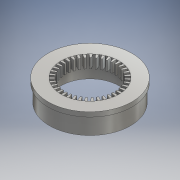
# Autodesk Inventor part: UR5 Wrist Rotation
Saved by Autodesk Inventor 2016 (Build 200138000, 138)
## iProperties
Created: 2017-12-25
Part Number: UR5 Wrist Rotation
Material: Aluminum 6061-AHC
Document SubType Name: Modeling
Designer: kornbot
Density: 2.7 g/cm^3
Appearance: Aluminum - Dark
Author: kornbot
Autodesk Inventor part; units mm, degrees
ref_plane "YZ Plane" through (0, 0, 0) normal (1, 0, 0) x (0, 1, 0)
ref_plane "XZ Plane" through (0, 0, 0) normal (0, 1, 0) x (-1, 0, 0)
ref_plane "XY Plane" through (0, 0, 0) normal (0, 0, 1) x (1, 0, 0)
sketch "Sketch1" plane through (0, 0, 0) normal (0, 0, 1) x (1, 0, 0)
  circle A0 centre (0, 0) radius 25.5
  circle A1 centre (0, 0) radius 35.6825
  dimension "d0" = 51
  dimension "d1" = 71.365
  constraints: 2 centre point, 2 coincident
  measures "d0" diameter of A0
  measures "d1" diameter of A1
extrude "Extrusion1" add sketch "Sketch1" along normal blind 19
sketch "Sketch2" plane through (0, 0, 19) normal (0, 0, 1) x (1, 0, 0)
  circle A0 centre (0, 0) radius 37
  circle A1 centre (0, 0) radius 35.6825
  dimension "d4" = 74
  constraints: 2 centre point, 2 coincident
  measures "d4" diameter of A0
extrude "Extrusion2" add sketch "Sketch2" against normal blind 4
sketch "Sketch3" plane through (0, 0, 19) normal (0, 0, 1) x (1, 0, 0)
  line L0 (-25.465862, -0.020576) -> (-21.481701, -0.020576)
  circle A0 centre (0, 0) radius 32.249031
  line L1 (-21.481701, -0.020576) -> (-21.481701, 0.604424)
  line L2 (-21.481701, -0.06479) -> (-21.481701, -0.68979)
  line L3 (-21.481701, -0.68979) -> (-25.479335, -1.026389)
  circle A1 centre (0, 0) radius 25.5
  line L4 (-21.481701, 0.604424) -> (-25.479335, 1.073894)
  line L5 (-25.479335, 1.073894) -> (-25.479335, -1.026389)
  line L6 (-25.479335, 1.073894) -> (-21.481701, 0.604424)
  line L7 (-21.481701, 0.604424) -> (-21.481701, -0.68979)
  line L8 (-21.481701, -0.68979) -> (-25.479335, -1.026389)
  line L9 (-25.479335, 1.073894) -> (-25.479335, -1.026389)
  line L10 (-25.479335, -1.026389) -> (-21.481701, -0.68979)
  line L11 (-21.481701, -0.68979) -> (-21.481701, 0.604424)
  line L12 (-21.481701, 0.604424) -> (-25.479335, 1.073894)
  line L13 (-21.300475, -2.849311) -> (-25.321649, -3.027185)
  line L14 (-21.200218, -3.466217) -> (-21.300475, -2.849311)
  line L15 (-21.300475, -2.849311) -> (-21.092869, -4.126765)
  line L16 (-21.092869, -4.126765) -> (-24.98474, -5.10027)
  line L17 (-25.321649, -3.027185) -> (-24.98474, -5.10027)
  line L18 (-20.567578, -6.229249) -> (-24.508146, -7.049862)
  line L19 (-20.369661, -6.822085) -> (-20.567578, -6.229249)
  line L20 (-20.567578, -6.229249) -> (-20.157742, -7.456858)
  line L21 (-20.157742, -7.456858) -> (-23.843054, -9.042057)
  line L22 (-24.508146, -7.049862) -> (-23.843054, -9.042057)
  line L23 (-19.301991, -9.447854) -> (-23.059894, -10.889951)
  line L24 (-19.011539, -10.001264) -> (-19.301991, -9.447854)
  line L25 (-19.301991, -9.447854) -> (-18.70054, -10.593823)
  line L26 (-18.70054, -10.593823) -> (-22.083844, -12.74966)
  line L27 (-23.059894, -10.889951) -> (-22.083844, -12.74966)
  line L28 (-17.536493, -12.421764) -> (-21.014404, -14.447997)
  line L29 (-17.161029, -12.921416) -> (-17.536493, -12.421764)
  line L30 (-17.536493, -12.421764) -> (-16.759005, -13.456414)
  line L31 (-16.759005, -13.456414) -> (-19.752675, -16.127053)
  line L32 (-21.014404, -14.447997) -> (-19.752675, -16.127053)
  line L33 (-15.316809, -15.073957) -> (-18.424651, -17.631846)
  line L34 (-14.866058, -15.506909) -> (-15.316809, -15.073957)
  line L35 (-15.316809, -15.073957) -> (-14.383419, -15.97049)
  line L36 (-14.383419, -15.97049) -> (-16.909922, -19.086763)
  line L37 (-18.424651, -17.631846) -> (-16.909922, -19.086763)
  line L38 (-12.700428, -17.335742) -> (-15.35771, -20.35904)
  line L39 (-12.186063, -17.690782) -> (-12.700428, -17.335742)
  line L40 (-12.700428, -17.335742) -> (-11.635311, -18.070939)
  line L41 (-11.635311, -18.070939) -> (-13.629211, -21.552137)
  line L42 (-15.35771, -20.35904) -> (-13.629211, -21.552137)
  line L43 (-9.755112, -19.14854) -> (-11.893012, -22.558946)
  line L44 (-9.190456, -19.416473) -> (-9.755112, -19.14854)
  line L45 (-9.755112, -19.14854) -> (-8.585854, -19.70336)
  line L46 (-8.585854, -19.70336) -> (-9.99551, -23.459322)
  line L47 (-11.893012, -22.558946) -> (-9.99551, -23.459322)
  line L48 (-6.557144, -20.465402) -> (-8.120291, -24.174587)
  line L49 (-5.95682, -20.639288) -> (-6.557144, -20.465402)
  line L50 (-6.557144, -20.465402) -> (-5.314029, -20.825475)
  line L51 (-5.314029, -20.825475) -> (-6.102931, -24.758922)
  line L52 (-8.120291, -24.174587) -> (-6.102931, -24.758922)
  line L53 (-3.18935, -21.25222) -> (-4.137259, -25.164119)
  line L54 (-2.568907, -21.327556) -> (-3.18935, -21.25222)
  line L55 (-3.18935, -21.25222) -> (-1.904572, -21.40822)
  line L56 (-1.904572, -21.40822) -> (-2.052289, -25.41728)
  line L57 (-4.137259, -25.164119) -> (-2.052289, -25.41728)
  line L58 (0.261048, -21.488617) -> (-0.047074, -25.501913)
  line L59 (0.885541, -21.463451) -> (0.261048, -21.488617)
  line L60 (0.261048, -21.488617) -> (1.554212, -21.436504)
  line L61 (1.554212, -21.436504) -> (2.051506, -25.417343)
  line L62 (-0.047074, -25.501913) -> (2.051506, -25.417343)
  line L63 (3.704684, -21.16847) -> (4.04433, -25.179221)
  line L64 (4.317053, -21.043454) -> (3.704684, -21.16847)
  line L65 (3.704684, -21.16847) -> (4.972742, -20.909594)
  line L66 (4.972742, -20.909594) -> (6.102168, -24.75911)
  line L67 (4.04433, -25.179221) -> (6.102168, -24.75911)
  line L68 (7.05237, -20.300071) -> (8.030988, -24.2044)
  line L69 (7.636756, -20.078443) -> (7.05237, -20.300071)
  line L70 (7.05237, -20.300071) -> (8.262481, -19.841137)
  line L71 (8.262481, -19.841137) -> (9.994787, -23.45963)
  line L72 (8.030988, -24.2044) -> (9.994787, -23.45963)
  line L73 (10.217404, -18.905911) -> (11.809648, -22.602699)
  line L74 (10.75867, -18.593411) -> (10.217404, -18.905911)
  line L75 (10.217404, -18.905911) -> (11.338226, -18.258804)
  line L76 (11.338226, -18.258804) -> (13.628546, -21.552557)
  line L77 (11.809648, -22.602699) -> (13.628546, -21.552557)
  line L78 (13.117813, -17.022097) -> (15.282444, -20.415599)
  line L79 (13.601941, -16.626819) -> (13.117813, -17.022097)
  line L80 (13.117813, -17.022097) -> (14.120317, -16.203578)
  line L81 (14.120317, -16.203578) -> (16.909334, -19.087285)
  line L82 (15.282444, -20.415599) -> (16.909334, -19.087285)
  line L83 (15.678477, -14.69742) -> (18.359433, -17.699746)
  line L84 (16.092929, -14.229601) -> (15.678477, -14.69742)
  line L85 (15.678477, -14.69742) -> (16.5367, -13.728688)
  line L86 (16.5367, -13.728688) -> (19.752178, -16.127661)
  line L87 (18.359433, -17.699746) -> (19.752178, -16.127661)
  line L88 (17.833077, -11.992088) -> (20.960922, -14.525479)
  line L89 (18.167118, -11.463844) -> (17.833077, -11.992088)
  line L90 (17.833077, -11.992088) -> (18.52479, -10.898231)
  line L91 (18.52479, -10.898231) -> (22.083451, -12.75034)
  line L92 (20.960922, -14.525479) -> (22.083451, -12.75034)
  line L93 (19.52581, -8.976167) -> (23.019534, -10.975009)
  line L94 (19.770789, -8.40118) -> (19.52581, -8.976167)
  line L95 (19.52581, -8.976167) -> (20.033098, -7.785517)
  line L96 (20.033098, -7.785517) -> (23.842775, -9.042792)
  line L97 (23.019534, -10.975009) -> (23.842775, -9.042792)
  line L98 (20.712834, -5.727768) -> (24.481952, -7.140293)
  line L99 (20.862406, -5.120929) -> (20.712834, -5.727768)
  line L100 (20.712834, -5.727768) -> (21.02256, -4.471162)
  line L101 (21.02256, -4.471162) -> (24.984583, -5.10104)
  line L102 (24.481952, -7.140293) -> (24.984583, -5.10104)
  line L103 (21.363407, -2.331022) -> (25.310301, -3.120647)
  line L104 (21.413698, -1.708049) -> (21.363407, -2.331022)
  line L105 (21.363407, -2.331022) -> (21.467548, -1.041005)
  line L106 (21.467548, -1.041005) -> (25.479304, -1.027174)
  line L107 (25.310301, -3.120647) -> (25.479304, -1.027174)
  line L108 (21.460679, 1.126095) -> (25.483126, 0.979823)
  line L109 (21.410387, 1.749069) -> (21.460679, 1.126095)
  line L110 (21.460679, 1.126095) -> (21.356538, 2.416112)
  line L111 (21.356538, 2.416112) -> (25.314124, 3.073295)
  line L112 (25.483126, 0.979823) -> (25.314124, 3.073295)
  line L113 (21.00213, 4.554047) -> (24.995952, 5.054915)
  line L114 (20.852558, 5.160886) -> (21.00213, 4.554047)
  line L115 (21.00213, 4.554047) -> (20.692404, 5.810654)
  line L116 (20.692404, 5.810654) -> (24.493321, 7.094168)
  line L117 (24.995952, 5.054915) -> (24.493321, 7.094168)
  line L118 (19.999637, 7.864052) -> (23.861395, 8.999088)
  line L119 (19.754658, 8.43904) -> (19.999637, 7.864052)
  line L120 (19.999637, 7.864052) -> (19.492349, 9.054702)
  line L121 (19.492349, 9.054702) -> (23.038155, 10.931305)
  line L122 (23.861395, 8.999088) -> (23.038155, 10.931305)
  line L123 (18.479165, 10.970382) -> (22.108841, 12.710189)
  line L124 (18.145123, 11.498626) -> (18.479165, 10.970382)
  line L125 (18.479165, 10.970382) -> (17.787452, 12.064239)
  line L126 (17.787452, 12.064239) -> (20.986312, 14.485328)
  line L127 (22.108841, 12.710189) -> (20.986312, 14.485328)
  line L128 (16.480091, 13.792585) -> (19.78368, 16.092103)
  line L129 (16.06564, 14.260404) -> (16.480091, 13.792585)
  line L130 (16.480091, 13.792585) -> (15.621869, 14.761318)
  line L131 (15.621869, 14.761318) -> (18.390935, 17.664188)
  line L132 (19.78368, 16.092103) -> (18.390935, 17.664188)
  line L133 (14.054192, 16.257567) -> (16.946131, 19.05724)
  line L134 (13.570064, 16.652846) -> (14.054192, 16.257567)
  line L135 (14.054192, 16.257567) -> (13.051688, 17.076087)
  line L136 (13.051688, 17.076087) -> (15.319242, 20.385554)
  line L137 (16.946131, 19.05724) -> (15.319242, 20.385554)
  line L138 (11.264297, 18.301487) -> (13.669687, 21.528805)
  line L139 (10.723031, 18.613987) -> (11.264297, 18.301487)
  line L140 (11.264297, 18.301487) -> (10.143475, 18.948594)
  line L141 (10.143475, 18.948594) -> (11.850789, 22.578946)
  line L142 (13.669687, 21.528805) -> (11.850789, 22.578946)
  line L143 (8.182662, 19.871408) -> (10.039205, 23.442784)
  line L144 (7.598277, 20.093036) -> (8.182662, 19.871408)
  line L145 (8.182662, 19.871408) -> (6.972551, 20.330342)
  line L146 (6.972551, 20.330342) -> (8.075407, 24.187555)
  line L147 (10.039205, 23.442784) -> (8.075407, 24.187555)
  line L148 (4.889101, 20.92667) -> (6.148713, 24.749608)
  line L149 (4.276732, 21.051686) -> (4.889101, 20.92667)
  line L150 (4.889101, 20.92667) -> (3.621042, 21.185546)
  line L151 (3.621042, 21.185546) -> (4.090876, 25.169719)
  line L152 (6.148713, 24.749608) -> (4.090876, 25.169719)
  line L153 (1.468914, 21.439942) -> (2.098973, 25.41543)
  line L154 (0.844421, 21.465108) -> (1.468914, 21.439942)
  line L155 (1.468914, 21.439942) -> (0.17575, 21.492055)
  line L156 (0.17575, 21.492055) -> (0.000393, 25.5)
  line L157 (2.098973, 25.41543) -> (0.000393, 25.5)
  line L158 (-1.989316, 21.397931) -> (-2.00513, 25.423006)
  line L159 (-2.609759, 21.322595) -> (-1.989316, 21.397931)
  line L160 (-1.989316, 21.397931) -> (-3.274094, 21.24193)
  line L161 (-3.274094, 21.24193) -> (-4.0901, 25.169845)
  line L162 (-2.00513, 25.423006) -> (-4.0901, 25.169845)
  line L163 (-5.396025, 20.801724) -> (-6.057301, 24.772139)
  line L164 (-5.996348, 20.627838) -> (-5.396025, 20.801724)
  line L165 (-5.396025, 20.801724) -> (-6.63914, 20.441651)
  line L166 (-6.63914, 20.441651) -> (-8.074661, 24.187804)
  line L167 (-6.057301, 24.772139) -> (-8.074661, 24.187804)
  line L168 (-8.662979, 19.666764) -> (-9.952591, 23.479687)
  line L169 (-9.227635, 19.398831) -> (-8.662979, 19.666764)
  line L170 (-8.662979, 19.666764) -> (-9.832237, 19.111944)
  line L171 (-9.832237, 19.111944) -> (-11.850093, 22.579311)
  line L172 (-9.952591, 23.479687) -> (-11.850093, 22.579311)
  line L173 (-11.705566, 18.022445) -> (-13.590115, 21.579123)
  line L174 (-12.219931, 17.667405) -> (-11.705566, 18.022445)
  line L175 (-11.705566, 18.022445) -> (-12.770683, 17.287248)
  line L176 (-12.770683, 17.287248) -> (-15.318614, 20.386027)
  line L177 (-13.590115, 21.579123) -> (-15.318614, 20.386027)
  line L178 (-14.444986, 15.911354) -> (-16.875661, 19.119672)
  line L179 (-14.895737, 15.478402) -> (-14.444986, 15.911354)
  line L180 (-14.444986, 15.911354) -> (-15.378376, 15.014821)
  line L181 (-15.378376, 15.014821) -> (-18.39039, 17.664754)
  line L182 (-16.875661, 19.119672) -> (-18.39039, 17.664754)
  line L183 (-16.810288, 13.388168) -> (-19.724137, 16.16503)
  line L184 (-17.185752, 12.888516) -> (-16.810288, 13.388168)
  line L185 (-16.810288, 13.388168) -> (-17.587777, 12.353518)
  line L186 (-17.587777, 12.353518) -> (-20.985865, 14.485974)
  line L187 (-19.724137, 16.16503) -> (-20.985865, 14.485974)
  line L188 (-18.740212, 10.518235) -> (-22.061767, 12.791724)
  line L189 (-19.030664, 9.964825) -> (-18.740212, 10.518235)
  line L190 (-18.740212, 10.518235) -> (-19.341663, 9.372266)
  line L191 (-19.341663, 9.372266) -> (-23.037818, 10.932015)
  line L192 (-22.061767, 12.791724) -> (-23.037818, 10.932015)
  line L193 (-20.184775, 7.375885) -> (-23.82801, 9.087118)
  line L194 (-20.382692, 6.78305) -> (-20.184775, 7.375885)
  line L195 (-20.184775, 7.375885) -> (-20.594611, 6.148276)
  line L196 (-20.594611, 6.148276) -> (-24.493103, 7.094923)
  line L197 (-23.82801, 9.087118) -> (-24.493103, 7.094923)
  line L198 (-21.106562, 4.042504) -> (-24.97712, 5.14716)
  line L199 (-21.206819, 3.425597) -> (-21.106562, 4.042504)
  line L200 (-21.106562, 4.042504) -> (-21.314169, 2.76505)
  line L201 (-21.314169, 2.76505) -> (-25.314029, 3.074075)
  line L202 (-24.97712, 5.14716) -> (-25.314029, 3.074075)
  point P0 (-21.193126, -3.509858)
  point P1 (-20.355659, -6.864023)
  point P2 (-18.990992, -10.040413)
  point P3 (-17.134468, -12.956762)
  point P4 (-14.834171, -15.537537)
  point P5 (-12.149676, -17.715898)
  point P6 (-9.150511, -19.435427)
  point P7 (-5.914352, -20.651589)
  point P8 (-2.525015, -21.332885)
  point P9 (0.929718, -21.461671)
  point P10 (4.360373, -21.03461)
  point P11 (7.678096, -20.062765)
  point P12 (10.79696, -18.571304)
  point P13 (13.636189, -16.598856)
  point P14 (16.122248, -14.196507)
  point P15 (18.190749, -11.426475)
  point P16 (19.788119, -8.360504)
  point P17 (20.872987, -5.078)
  point P18 (21.417256, -1.663979)
  point P19 (21.406829, 1.793139)
  point P20 (20.841977, 5.203815)
  point P21 (19.737328, 8.479715)
  point P22 (18.121493, 11.535995)
  point P23 (16.03632, 14.293499)
  point P24 (13.535816, 16.680809)
  point P25 (10.684741, 18.636094)
  point P26 (7.556936, 20.108714)
  point P27 (4.233411, 21.06053)
  point P28 (0.800243, 21.466888)
  point P29 (-2.653651, 21.317266)
  point P30 (-6.038816, 20.615537)
  point P31 (-9.26758, 19.379877)
  point P32 (-12.256318, 17.642289)
  point P33 (-14.927624, 15.447774)
  point P34 (-17.212313, 12.85317)
  point P35 (-19.051211, 9.925676)
  point P36 (-20.396693, 6.741111)
  point P37 (-21.213912, 3.381956)
  dimension "d13" = 0.625
  dimension "d14" = 0.625
  dimension "d17" = 360
  constraints: 406 end point, 78 point on line, 5 collinear, 2 vertical, 1 centre point, 1 coincident, 1 horizontal, 432 other
  measures "d13" distance of L0.end L1.end
  measures "d14" distance of L2.start L2.end
sketch "Sketch3 outline for Extrusion3" plane through (0, 0, 19) normal (0, 0, 1) x (1, 0, 0)
  circle A0 centre (0, 0) radius 32.249031
  arc A1 (25.314124, -3.073295) -> (25.479304, -1.027174) centre (0, 0) ccw
  line L0 (25.314124, -3.073295) -> (25.479304, -1.027174)
  line L1 (25.479304, -1.027174) -> (21.467548, -1.041005)
  line L2 (21.467548, -1.041005) -> (21.363407, -2.331022)
  line L3 (21.363407, -2.331022) -> (25.308377, -3.120262)
  arc A2 (24.984583, -5.10104) -> (25.308377, -3.120262) centre (0, 0) ccw
  line L4 (24.984583, -5.10104) -> (21.02256, -4.471162)
  line L5 (21.02256, -4.471162) -> (20.712834, -5.727768)
  line L6 (20.712834, -5.727768) -> (24.480115, -7.139604)
  arc A3 (23.842775, -9.042792) -> (24.480115, -7.139604) centre (0, 0) ccw
  line L7 (23.842775, -9.042792) -> (20.033098, -7.785517)
  line L8 (20.033098, -7.785517) -> (19.52581, -8.976167)
  line L9 (19.52581, -8.976167) -> (23.017831, -10.974035)
  arc A4 (22.083451, -12.75034) -> (23.017831, -10.974035) centre (0, 0) ccw
  line L10 (22.083451, -12.75034) -> (18.52479, -10.898231)
  line L11 (18.52479, -10.898231) -> (17.833077, -11.992088)
  line L12 (17.833077, -11.992088) -> (20.959397, -14.524244)
  arc A5 (19.752178, -16.127661) -> (20.959397, -14.524244) centre (0, 0) ccw
  line L13 (19.752178, -16.127661) -> (16.5367, -13.728688)
  line L14 (16.5367, -13.728688) -> (15.678477, -14.69742)
  line L15 (15.678477, -14.69742) -> (18.358126, -17.698283)
  arc A6 (16.909334, -19.087285) -> (18.358126, -17.698283) centre (0, 0) ccw
  line L16 (16.909334, -19.087285) -> (14.120317, -16.203578)
  line L17 (14.120317, -16.203578) -> (13.117813, -17.022097)
  line L18 (13.117813, -17.022097) -> (15.281389, -20.413945)
  arc A7 (13.628546, -21.552557) -> (15.281389, -20.413945) centre (0, 0) ccw
  line L19 (13.628546, -21.552557) -> (11.338226, -18.258804)
  line L20 (11.338226, -18.258804) -> (10.217404, -18.905911)
  line L21 (10.217404, -18.905911) -> (11.808872, -22.600897)
  arc A8 (9.994787, -23.45963) -> (11.808872, -22.600897) centre (0, 0) ccw
  line L22 (9.994787, -23.45963) -> (8.262481, -19.841137)
  line L23 (8.262481, -19.841137) -> (7.05237, -20.300071)
  line L24 (7.05237, -20.300071) -> (8.030511, -24.202498)
  arc A9 (6.102168, -24.75911) -> (8.030511, -24.202498) centre (0, 0) ccw
  line L25 (6.102168, -24.75911) -> (4.972742, -20.909594)
  line L26 (4.972742, -20.909594) -> (3.704684, -21.16847)
  line L27 (3.704684, -21.16847) -> (4.044165, -25.177266)
  arc A10 (2.051506, -25.417343) -> (4.044165, -25.177266) centre (0, 0) ccw
  line L28 (2.051506, -25.417343) -> (1.554212, -21.436504)
  line L29 (1.554212, -21.436504) -> (0.261048, -21.488617)
  line L30 (0.261048, -21.488617) -> (-0.046924, -25.499957)
  arc A11 (-2.052289, -25.41728) -> (-0.046924, -25.499957) centre (0, 0) ccw
  line L31 (-2.052289, -25.41728) -> (-1.904572, -21.40822)
  line L32 (-1.904572, -21.40822) -> (-3.18935, -21.25222)
  line L33 (-3.18935, -21.25222) -> (-4.136797, -25.162212)
  arc A12 (-6.102931, -24.758922) -> (-4.136797, -25.162212) centre (0, 0) ccw
  line L34 (-6.102931, -24.758922) -> (-5.314029, -20.825475)
  line L35 (-5.314029, -20.825475) -> (-6.557144, -20.465402)
  line L36 (-6.557144, -20.465402) -> (-8.119529, -24.172779)
  arc A13 (-9.99551, -23.459322) -> (-8.119529, -24.172779) centre (0, 0) ccw
  line L37 (-9.99551, -23.459322) -> (-8.585854, -19.70336)
  line L38 (-8.585854, -19.70336) -> (-9.755112, -19.14854)
  line L39 (-9.755112, -19.14854) -> (-11.89197, -22.557284)
  arc A14 (-13.629211, -21.552137) -> (-11.89197, -22.557284) centre (0, 0) ccw
  line L40 (-13.629211, -21.552137) -> (-11.635311, -18.070939)
  line L41 (-11.635311, -18.070939) -> (-12.700428, -17.335742)
  line L42 (-12.700428, -17.335742) -> (-15.356415, -20.357567)
  arc A15 (-16.909922, -19.086763) -> (-15.356415, -20.357567) centre (0, 0) ccw
  line L43 (-16.909922, -19.086763) -> (-14.383419, -15.97049)
  line L44 (-14.383419, -15.97049) -> (-15.316809, -15.073957)
  line L45 (-15.316809, -15.073957) -> (-18.423136, -17.6306)
  arc A16 (-19.752675, -16.127053) -> (-18.423136, -17.6306) centre (0, 0) ccw
  line L46 (-19.752675, -16.127053) -> (-16.759005, -13.456414)
  line L47 (-16.759005, -13.456414) -> (-17.536493, -12.421764)
  line L48 (-17.536493, -12.421764) -> (-21.012709, -14.447009)
  arc A17 (-22.083844, -12.74966) -> (-21.012709, -14.447009) centre (0, 0) ccw
  line L49 (-22.083844, -12.74966) -> (-18.70054, -10.593823)
  line L50 (-18.70054, -10.593823) -> (-19.301991, -9.447854)
  line L51 (-19.301991, -9.447854) -> (-23.058063, -10.889249)
  arc A18 (-23.843054, -9.042057) -> (-23.058063, -10.889249) centre (0, 0) ccw
  line L52 (-23.843054, -9.042057) -> (-20.157742, -7.456858)
  line L53 (-20.157742, -7.456858) -> (-20.567578, -6.229249)
  line L54 (-20.567578, -6.229249) -> (-24.506225, -7.049462)
  arc A19 (-24.98474, -5.10027) -> (-24.506225, -7.049462) centre (0, 0) ccw
  line L55 (-24.98474, -5.10027) -> (-21.092869, -4.126765)
  line L56 (-21.092869, -4.126765) -> (-21.300475, -2.849311)
  line L57 (-21.300475, -2.849311) -> (-25.319689, -3.027099)
  arc A20 (-25.479335, -1.026389) -> (-25.319689, -3.027099) centre (0, 0) ccw
  line L58 (-25.479335, -1.026389) -> (-21.481701, -0.68979)
  line L59 (-21.481701, -0.68979) -> (-21.481701, 0.604424)
  line L60 (-21.481701, 0.604424) -> (-25.477387, 1.073665)
  arc A21 (-25.314029, 3.074075) -> (-25.477387, 1.073665) centre (0, 0) ccw
  line L61 (-25.314029, 3.074075) -> (-21.314169, 2.76505)
  line L62 (-21.314169, 2.76505) -> (-21.106562, 4.042504)
  line L63 (-21.106562, 4.042504) -> (-24.975233, 5.146622)
  arc A22 (-24.493103, 7.094923) -> (-24.975233, 5.146622) centre (0, 0) ccw
  line L64 (-24.493103, 7.094923) -> (-20.594611, 6.148276)
  line L65 (-20.594611, 6.148276) -> (-20.184775, 7.375885)
  line L66 (-20.184775, 7.375885) -> (-23.826234, 9.086284)
  arc A23 (-23.037818, 10.932015) -> (-23.826234, 9.086284) centre (0, 0) ccw
  line L67 (-23.037818, 10.932015) -> (-19.341663, 9.372266)
  line L68 (-19.341663, 9.372266) -> (-18.740212, 10.518235)
  line L69 (-18.740212, 10.518235) -> (-22.060149, 12.790615)
  arc A24 (-20.985865, 14.485974) -> (-22.060149, 12.790615) centre (0, 0) ccw
  line L70 (-20.985865, 14.485974) -> (-17.587777, 12.353518)
  line L71 (-17.587777, 12.353518) -> (-16.810288, 13.388168)
  line L72 (-16.810288, 13.388168) -> (-19.722716, 16.163677)
  arc A25 (-18.39039, 17.664754) -> (-19.722716, 16.163677) centre (0, 0) ccw
  line L73 (-18.39039, 17.664754) -> (-15.378376, 15.014821)
  line L74 (-15.378376, 15.014821) -> (-14.444986, 15.911354)
  line L75 (-14.444986, 15.911354) -> (-16.874476, 19.118108)
  arc A26 (-15.318614, 20.386027) -> (-16.874476, 19.118108) centre (0, 0) ccw
  line L76 (-15.318614, 20.386027) -> (-12.770683, 17.287248)
  line L77 (-12.770683, 17.287248) -> (-11.705566, 18.022445)
  line L78 (-11.705566, 18.022445) -> (-13.589196, 21.57739)
  arc A27 (-11.850093, 22.579311) -> (-13.589196, 21.57739) centre (0, 0) ccw
  line L79 (-11.850093, 22.579311) -> (-9.832237, 19.111944)
  line L80 (-9.832237, 19.111944) -> (-8.662979, 19.666764)
  line L81 (-8.662979, 19.666764) -> (-9.951963, 23.477829)
  arc A28 (-8.074661, 24.187804) -> (-9.951963, 23.477829) centre (0, 0) ccw
  line L82 (-8.074661, 24.187804) -> (-6.63914, 20.441651)
  line L83 (-6.63914, 20.441651) -> (-5.396025, 20.801724)
  line L84 (-5.396025, 20.801724) -> (-6.056979, 24.770204)
  arc A29 (-4.0901, 25.169845) -> (-6.056979, 24.770204) centre (0, 0) ccw
  line L85 (-4.0901, 25.169845) -> (-3.274094, 21.24193)
  line L86 (-3.274094, 21.24193) -> (-1.989316, 21.397931)
  line L87 (-1.989316, 21.397931) -> (-2.005123, 25.421044)
  arc A30 (0.000393, 25.5) -> (-2.005123, 25.421044) centre (0, 0) ccw
  line L88 (0.000393, 25.5) -> (0.17575, 21.492055)
  line L89 (0.17575, 21.492055) -> (1.468914, 21.439942)
  line L90 (1.468914, 21.439942) -> (2.098666, 25.413493)
  arc A31 (4.090876, 25.169719) -> (2.098666, 25.413493) centre (0, 0) ccw
  line L91 (4.090876, 25.169719) -> (3.621042, 21.185546)
  line L92 (3.621042, 21.185546) -> (4.889101, 20.92667)
  line L93 (4.889101, 20.92667) -> (6.148099, 24.747745)
  arc A32 (8.075407, 24.187555) -> (6.148099, 24.747745) centre (0, 0) ccw
  line L94 (8.075407, 24.187555) -> (6.972551, 20.330342)
  line L95 (6.972551, 20.330342) -> (8.182662, 19.871408)
  line L96 (8.182662, 19.871408) -> (10.0383, 23.441044)
  arc A33 (11.850789, 22.578946) -> (10.0383, 23.441044) centre (0, 0) ccw
  line L97 (11.850789, 22.578946) -> (10.143475, 18.948594)
  line L98 (10.143475, 18.948594) -> (11.264297, 18.301487)
  line L99 (11.264297, 18.301487) -> (13.668515, 21.527232)
  arc A34 (15.319242, 20.385554) -> (13.668515, 21.527232) centre (0, 0) ccw
  line L100 (15.319242, 20.385554) -> (13.051688, 17.076087)
  line L101 (13.051688, 17.076087) -> (14.054192, 16.257567)
  line L102 (14.054192, 16.257567) -> (16.944722, 19.055876)
  arc A35 (18.390935, 17.664188) -> (16.944722, 19.055876) centre (0, 0) ccw
  line L103 (18.390935, 17.664188) -> (15.621869, 14.761318)
  line L104 (15.621869, 14.761318) -> (16.480091, 13.792585)
  line L105 (16.480091, 13.792585) -> (19.78207, 16.090982)
  arc A36 (20.986312, 14.485328) -> (19.78207, 16.090982) centre (0, 0) ccw
  line L106 (20.986312, 14.485328) -> (17.787452, 12.064239)
  line L107 (17.787452, 12.064239) -> (18.479165, 10.970382)
  line L108 (18.479165, 10.970382) -> (22.107072, 12.709341)
  arc A37 (23.038155, 10.931305) -> (22.107072, 12.709341) centre (0, 0) ccw
  line L109 (23.038155, 10.931305) -> (19.492349, 9.054702)
  line L110 (19.492349, 9.054702) -> (19.999637, 7.864052)
  line L111 (19.999637, 7.864052) -> (23.859513, 8.998535)
  arc A38 (24.493321, 7.094168) -> (23.859513, 8.998535) centre (0, 0) ccw
  line L112 (24.493321, 7.094168) -> (20.692404, 5.810654)
  line L113 (20.692404, 5.810654) -> (21.00213, 4.554047)
  line L114 (21.00213, 4.554047) -> (24.994005, 5.054671)
  arc A39 (25.314124, 3.073295) -> (24.994005, 5.054671) centre (0, 0) ccw
  line L115 (25.314124, 3.073295) -> (21.356538, 2.416112)
  line L116 (21.356538, 2.416112) -> (21.460679, 1.126095)
  line L117 (21.460679, 1.126095) -> (25.481166, 0.979894)
  arc A40 (25.481166, 0.979894) -> (25.479304, -1.027174) centre (0, 0) cw
  arc A41 (24.493321, -7.094168) -> (24.984583, -5.10104) centre (0, 0) ccw
  line L118 (24.493321, -7.094168) -> (24.984583, -5.10104)
  arc A42 (23.038155, -10.931305) -> (23.842775, -9.042792) centre (0, 0) ccw
  line L119 (23.038155, -10.931305) -> (23.842775, -9.042792)
  arc A43 (20.986312, -14.485328) -> (22.083451, -12.75034) centre (0, 0) ccw
  line L120 (20.986312, -14.485328) -> (22.083451, -12.75034)
  arc A44 (18.390935, -17.664188) -> (19.752178, -16.127661) centre (0, 0) ccw
  line L121 (18.390935, -17.664188) -> (19.752178, -16.127661)
  arc A45 (15.319242, -20.385554) -> (16.909334, -19.087285) centre (0, 0) ccw
  line L122 (15.319242, -20.385554) -> (16.909334, -19.087285)
  arc A46 (11.850789, -22.578946) -> (13.628546, -21.552557) centre (0, 0) ccw
  line L123 (11.850789, -22.578946) -> (13.628546, -21.552557)
  arc A47 (8.075407, -24.187555) -> (9.994787, -23.45963) centre (0, 0) ccw
  line L124 (8.075407, -24.187555) -> (9.994787, -23.45963)
  arc A48 (4.090876, -25.169719) -> (6.102168, -24.75911) centre (0, 0) ccw
  line L125 (4.090876, -25.169719) -> (6.102168, -24.75911)
  arc A49 (0.000393, -25.5) -> (2.051506, -25.417343) centre (0, 0) ccw
  line L126 (0.000393, -25.5) -> (2.051506, -25.417343)
  arc A50 (-4.0901, -25.169845) -> (-2.052289, -25.41728) centre (0, 0) ccw
  line L127 (-4.0901, -25.169845) -> (-2.052289, -25.41728)
  arc A51 (-8.074661, -24.187804) -> (-6.102931, -24.758922) centre (0, 0) ccw
  line L128 (-8.074661, -24.187804) -> (-6.102931, -24.758922)
  arc A52 (-11.850093, -22.579311) -> (-9.99551, -23.459322) centre (0, 0) ccw
  line L129 (-11.850093, -22.579311) -> (-9.99551, -23.459322)
  arc A53 (-15.318614, -20.386027) -> (-13.629211, -21.552137) centre (0, 0) ccw
  line L130 (-15.318614, -20.386027) -> (-13.629211, -21.552137)
  arc A54 (-18.39039, -17.664754) -> (-16.909922, -19.086763) centre (0, 0) ccw
  line L131 (-18.39039, -17.664754) -> (-16.909922, -19.086763)
  arc A55 (-20.985865, -14.485974) -> (-19.752675, -16.127053) centre (0, 0) ccw
  line L132 (-20.985865, -14.485974) -> (-19.752675, -16.127053)
  arc A56 (-23.037818, -10.932015) -> (-22.083844, -12.74966) centre (0, 0) ccw
  line L133 (-23.037818, -10.932015) -> (-22.083844, -12.74966)
  arc A57 (-24.493103, -7.094923) -> (-23.843054, -9.042057) centre (0, 0) ccw
  line L134 (-24.493103, -7.094923) -> (-23.843054, -9.042057)
  arc A58 (-25.314029, -3.074075) -> (-24.98474, -5.10027) centre (0, 0) ccw
  line L135 (-25.314029, -3.074075) -> (-24.98474, -5.10027)
  arc A59 (-25.479335, 1.026389) -> (-25.479335, -1.026389) centre (0, 0) ccw
  line L136 (-25.479335, 1.026389) -> (-25.479335, -1.026389)
  arc A60 (-24.98474, 5.10027) -> (-25.314029, 3.074075) centre (0, 0) ccw
  line L137 (-24.98474, 5.10027) -> (-25.314029, 3.074075)
  arc A61 (-23.843054, 9.042057) -> (-24.493103, 7.094923) centre (0, 0) ccw
  line L138 (-23.843054, 9.042057) -> (-24.493103, 7.094923)
  arc A62 (-22.083844, 12.74966) -> (-23.037818, 10.932015) centre (0, 0) ccw
  line L139 (-22.083844, 12.74966) -> (-23.037818, 10.932015)
  arc A63 (-19.752675, 16.127053) -> (-20.985865, 14.485974) centre (0, 0) ccw
  line L140 (-19.752675, 16.127053) -> (-20.985865, 14.485974)
  arc A64 (-16.909922, 19.086763) -> (-18.39039, 17.664754) centre (0, 0) ccw
  line L141 (-16.909922, 19.086763) -> (-18.39039, 17.664754)
  arc A65 (-13.629211, 21.552137) -> (-15.318614, 20.386027) centre (0, 0) ccw
  line L142 (-13.629211, 21.552137) -> (-15.318614, 20.386027)
  arc A66 (-9.99551, 23.459322) -> (-11.850093, 22.579311) centre (0, 0) ccw
  line L143 (-9.99551, 23.459322) -> (-11.850093, 22.579311)
  arc A67 (-6.102931, 24.758922) -> (-8.074661, 24.187804) centre (0, 0) ccw
  line L144 (-6.102931, 24.758922) -> (-8.074661, 24.187804)
  arc A68 (-2.052289, 25.41728) -> (-4.0901, 25.169845) centre (0, 0) ccw
  line L145 (-2.052289, 25.41728) -> (-4.0901, 25.169845)
  arc A69 (2.051506, 25.417343) -> (0.000393, 25.5) centre (0, 0) ccw
  line L146 (2.051506, 25.417343) -> (0.000393, 25.5)
  arc A70 (6.102168, 24.75911) -> (4.090876, 25.169719) centre (0, 0) ccw
  line L147 (6.102168, 24.75911) -> (4.090876, 25.169719)
  arc A71 (9.994787, 23.45963) -> (8.075407, 24.187555) centre (0, 0) ccw
  line L148 (9.994787, 23.45963) -> (8.075407, 24.187555)
  arc A72 (13.628546, 21.552557) -> (11.850789, 22.578946) centre (0, 0) ccw
  line L149 (13.628546, 21.552557) -> (11.850789, 22.578946)
  arc A73 (16.909334, 19.087285) -> (15.319242, 20.385554) centre (0, 0) ccw
  line L150 (16.909334, 19.087285) -> (15.319242, 20.385554)
  arc A74 (19.752178, 16.127661) -> (18.390935, 17.664188) centre (0, 0) ccw
  line L151 (19.752178, 16.127661) -> (18.390935, 17.664188)
  arc A75 (22.083451, 12.75034) -> (20.986312, 14.485328) centre (0, 0) ccw
  line L152 (22.083451, 12.75034) -> (20.986312, 14.485328)
  arc A76 (23.842775, 9.042792) -> (23.038155, 10.931305) centre (0, 0) ccw
  line L153 (23.842775, 9.042792) -> (23.038155, 10.931305)
  arc A77 (24.984583, 5.10104) -> (24.493321, 7.094168) centre (0, 0) ccw
  line L154 (24.984583, 5.10104) -> (24.493321, 7.094168)
  arc A78 (25.479304, 1.027174) -> (25.314124, 3.073295) centre (0, 0) ccw
  line L155 (25.479304, 1.027174) -> (25.314124, 3.073295)
extrude "Extrusion3" add sketch "Sketch3 outline for Extrusion3" against normal blind 8.5
body "Solid1"
